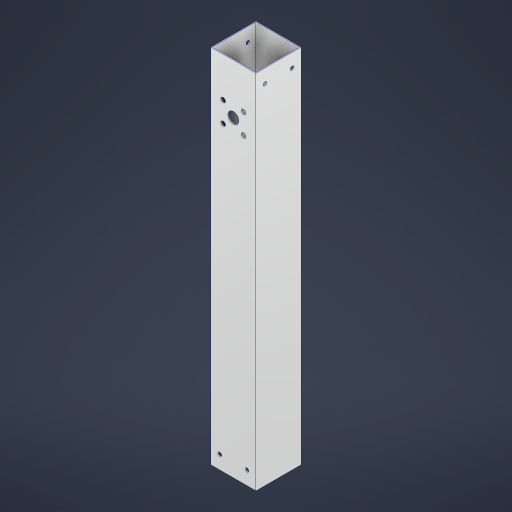
# Autodesk Inventor part: End-Link
Saved by Autodesk Inventor 2023 (Build 270158000, 158)
## iProperties
Created: 2023-08-12
Part Number: End-Link
Material: Aluminum 6061
Document SubType Name: Modeling
Designer: Abhinav
Density: 2.7 g/cm^3
Appearance: Aluminum - Flat
Author: Abhinav
Autodesk Inventor part; units mm, degrees
ref_plane "YZ Plane" through (0, 0, 0) normal (1, 0, 0) x (0, 1, 0)
ref_plane "XZ Plane" through (0, 0, 0) normal (0, 1, 0) x (-1, 0, 0)
ref_plane "XY Plane" through (0, 0, 0) normal (0, 0, 1) x (1, 0, 0)
sketch "Sketch1" plane through (0, 0, 0) normal (0, 1, 0) x (-1, 0, 0)
  line L0 (25, 25) -> (-25, 25)
  line L1 (-25, 25) -> (-25, -25)
  line L2 (-25, -25) -> (25, -25)
  line L3 (25, -25) -> (25, 25)
  line L4 (25, 25) -> (-25, -25) construction
  line L5 (-25, 25) -> (25, -25) construction
  line L6 (24, 24) -> (-24, 24)
  line L7 (-24, 24) -> (-24, -24)
  line L8 (-24, -24) -> (24, -24)
  line L9 (24, -24) -> (24, 24)
  line L10 (24, 24) -> (-24, -24) construction
  line L11 (-24, 24) -> (24, -24) construction
  point P0 (0, 0)
  dimension "d0" = 50
  dimension "d2" = 48
  constraints: 24 end point, 4 midpoint, 4 parallel, 4 perpendicular, 2 horizontal
  measures "d0" distance of L2.end L1.end
  measures "d2" distance of L8.end L7.end
extrude "Extrusion1" add sketch "Sketch1" along normal blind 400
sketch "Sketch3" plane through (25, 0, -25) normal (0, 0, -1) x (-1, 0, 0)
  line L0 (50, 0) -> (50, 400) projected
  line L1 (0, 0) -> (0, 400) projected
  line L2 (50, 0) -> (50, 400) projected
  line L3 (0, 400) -> (50, 400)
  line L4 (50, 400) -> (50, 370)
  line L5 (50, 370) -> (0, 370)
  line L6 (0, 370) -> (0, 400)
  line L7 (0, 400) -> (50, 370) construction
  line L8 (25, 385) -> (40, 385) construction
  line L9 (25, 385) -> (10, 385) construction
  line L10 (0, 30) -> (50, 30)
  line L11 (50, 30) -> (50, 0)
  line L12 (50, 0) -> (0, 0)
  line L13 (0, 0) -> (0, 30)
  line L14 (0, 30) -> (50, 0) construction
  circle A0 centre (40, 15) radius 2
  line L15 (25, 15) -> (40, 15) construction
  line L16 (25, 15) -> (10, 15) construction
  circle A1 centre (10, 15) radius 2
  line L17 (25, 385) -> (25, 345) construction
  circle A2 centre (25, 345) radius 6
  line L18 (25, 345) -> (36.3137, 333.6863) construction
  line L19 (0, 0) -> (16, 0) construction
  line L20 (25, 345) -> (13.6863, 356.3137) construction
  circle A3 centre (36.3137, 333.6863) radius 2.5
  circle A4 centre (13.6863, 356.3137) radius 2.5
  circle A5 centre (36.3137, 356.3137) radius 2.5
  circle A6 centre (13.6863, 333.6863) radius 2.5
  dimension "d28" = 30
  dimension "d30" = 15
  dimension "d31" = 15
  dimension "d33" = 30
  dimension "d34" = 4
  dimension "d35" = 15
  dimension "d36" = 15
  dimension "d37" = 4
  dimension "d38" = 40
  dimension "d61" = 12
  dimension "d64" = 16
  dimension "d65" = 5
  constraints: 36 end point, 7 centre point, 5 coincident, 5 horizontal, 4 parallel, 3 point on line, 2 equal length, 2 perpendicular, 1 equal radius, 1 vertical
  measures "d28" distance of L3.end L4.end
  measures "d30" distance of L8.start L8.end
  measures "d31" distance of L9.start L9.end
  measures "d33" distance of L10.end L11.end
  measures "d34" diameter of A0
  measures "d35" distance of L15.start L15.end
  measures "d36" distance of L16.start L16.end
  measures "d37" diameter of A1
  measures "d38" distance of L9.start L17.end
  measures "d61" diameter of A2
  measures "d64" distance of L18.start L20.end
  measures "d65" diameter of A3
extrude "Extrusion3" cut sketch "Sketch3" against normal blind 50 contours A0 | A1 | A2 | A3 | A4 | A5 | A6
sketch "Sketch5" plane through (25, 0, 25) normal (1, 0, 0) x (0, 0, -1)
  line L0 (0, 400) -> (50, 400)
  line L1 (50, 400) -> (50, 370)
  line L2 (50, 370) -> (0, 370)
  line L3 (0, 370) -> (0, 400)
  line L4 (0, 400) -> (50, 370) construction
  circle A0 centre (40, 385) radius 2
  line L5 (25, 385) -> (40, 385) construction
  line L6 (25, 385) -> (10, 385) construction
  circle A1 centre (10, 385) radius 2
  point P0 (25, 0)
  dimension "d40" = 30
  dimension "d41" = 4
  dimension "d42" = 15
  dimension "d43" = 15
  dimension "d44" = 4
  constraints: 14 end point, 2 centre point, 2 horizontal, 2 parallel, 1 coincident, 1 perpendicular, 1 point on line
  measures "d40" distance of L1.start L1.end
  measures "d41" diameter of A0
  measures "d42" distance of L5.start L5.end
  measures "d43" distance of L6.start L6.end
  measures "d44" diameter of A1
extrude "Extrusion5" cut sketch "Sketch5" against normal blind 50 contours A0 | A1
body "Solid1"
